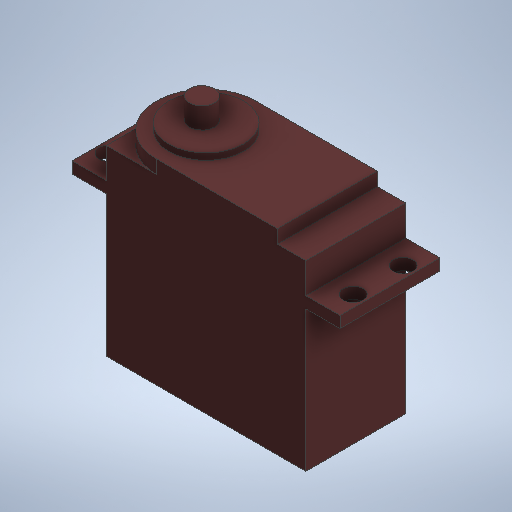
# Autodesk Inventor part: 996R모터
Saved by Autodesk Inventor 2025.2 (Build 292293000, 293)
## iProperties
Created: 2024-03-19
Part Number: 996R모터
Material: 일반
Document SubType Name: Modeling
Designer: USER
Density: 1 g/cm^3
Appearance: 기본값
Author: USER
## iProperties of the stored document 996R모터_3D 인쇄.ipt
Created: 2024-04-18
Part Number: 996R모터_3D 인쇄
Material: 일반
Document SubType Name: Modeling
Designer: USER
Density: 1 g/cm^3
Appearance: 기본값
Author: USER
Autodesk Inventor part; units mm, degrees
ref_plane "YZ Plane" through (0, 0, 0) normal (1, 0, 0) x (0, 1, 0)
ref_plane "XZ Plane" through (0, 0, 0) normal (0, 1, 0) x (-1, 0, 0)
ref_plane "XY Plane" through (0, 0, 0) normal (0, 0, 1) x (1, 0, 0)
sketch "스케치1" plane through (0, 0, 0) normal (0, 0, 1) x (1, 0, 0)
  line L0 (0, 0) -> (40, 0)
  line L1 (40, 0) -> (40, 36.6)
  line L2 (40, 36.6) -> (0, 36.6)
  line L3 (0, 36.6) -> (0, 0)
  dimension "d0" = 40
  dimension "d1" = 36.6
  constraints: 8 end point, 2 parallel, 1 horizontal, 1 perpendicular
  measures "d0" distance of L2.end L1.end
  measures "d1" distance of L0.end L1.end
extrude "돌출1" add sketch "스케치1" along normal blind 20
sketch "스케치2" plane through (0, 0, 20) normal (0, 0, 1) x (1, 0, 0)
  line L0 (40, 0) -> (40, 36.6) projected
  line L1 (40, 30.5) -> (46.85, 30.5)
  line L2 (46.85, 30.5) -> (46.85, 28.2)
  line L3 (46.85, 28.2) -> (40, 28.2)
  line L4 (40, 28.2) -> (40, 30.5)
  line L5 (0, 30.5) -> (-6.85, 30.5)
  line L6 (-6.85, 30.5) -> (-6.85, 28.2)
  line L7 (-6.85, 28.2) -> (0, 28.2)
  line L8 (0, 28.2) -> (0, 30.5)
  line L9 (0, 0) -> (40, 0) projected
  line L10 (0, 36.6) -> (0, 0) projected
  point P0 (40, 28.2)
  point P1 (0, 29.35)
  dimension "d4" = 6.85
  dimension "d5" = 6.85
  dimension "d6" = 2.3
  dimension "d7" = 2.3
  dimension "d8" = 30.5
  dimension "d9" = 30.5
  constraints: 16 end point, 4 parallel, 2 horizontal, 2 perpendicular, 2 point on line, 1 midpoint
  measures "d4" distance of L2.end L3.end
  measures "d5" distance of L7.end L6.end
  measures "d6" distance between parallel lines of L3 L1
  measures "d7" distance between parallel lines of L7 L5
  measures "d8" distance between parallel lines of L9 L1
  measures "d9" distance between parallel lines of L9 L5
extrude "돌출2" add sketch "스케치2" against normal blind 20
sketch "스케치3" plane through (0, 36.6, 0) normal (0, 1, 0) x (1, 0, 0)
  line L0 (40, 0) -> (0, 0) projected
  line L1 (0, 0) -> (0, -20) projected
  line L2 (40, -20) -> (0, -20) projected
  line L3 (40, 0) -> (40, -20) projected
  circle A0 centre (10, -10) radius 10
  line L4 (0, 0) -> (0, -20) projected
  line L5 (0, -20) -> (34.3, -20)
  line L6 (34.3, -20) -> (34.3, 0)
  line L7 (34.3, 0) -> (0, 0)
  line L8 (0, 0) -> (0, -20)
  line L9 (40, -20) -> (0, -20) projected
  point P0 (10, -20)
  point P1 (10, 0)
  dimension "d12" = 34.3
  constraints: 8 end point, 3 tangent, 2 parallel, 1 centre point, 1 horizontal, 1 perpendicular, 1 point on line
  measures "d12" distance of L7.end L6.end
extrude "돌출3" add sketch "스케치3" along normal blind 2.7 contours L6 L2 A0 L0 | A0
sketch "스케치4" plane through (0, 39.3, 0) normal (0, 1, 0) x (1, 0, 0)
  circle A0 centre (9.15, -10) radius 2.5
  arc A1 (10, 0) -> (10, -20) centre (10, -10) ccw projected
  line L0 (-6.85, -20) -> (-6.85, 0) projected
  point P0 (0, 0)
  point P1 (0, -10)
  point P2 (11.638, -9.755)
  point P3 (0, -10)
  point P4 (0, -10)
  dimension "d15" = 5
  dimension "d23" = 16
  constraints: 3 point on circle, 1 horizontal alignment, 3 other
  measures "d23" distance from line of L0 point (9.15, -10)
extrude "돌출4" add sketch "스케치4" along normal blind 5.5
sketch "스케치5" plane through (0, 39.3, 0) normal (0, 1, 0) x (1, 0, 0)
  circle A0 centre (9.15, -10) radius 2.5 projected
  line L0 (10, -20) -> (34.3, -20) projected
  line L1 (34.3, -20) -> (34.3, 0) projected
  line L2 (34.3, 0) -> (10, 0) projected
  arc A1 (10, 0) -> (10, -20) centre (10, -10) ccw projected
  circle A2 centre (10, -10) radius 7.5
  point P0 (0, 0)
  dimension "d20" = 15
  constraints: 1 centre point, 1 coincident
  measures "d20" diameter of A2
sketch "스케치6" plane through (0, 0, 20) normal (0, 0, 1) x (1, 0, 0)
  point P0 (0, 0)
extrude "돌출5" add sketch "스케치5" along normal blind 1.3 contours A2
sketch "스케치18" plane through (0, 39.3, 0) normal (0, 1, 0) x (1, 0, 0)
  point P0 (0, 0)
sketch "스케치19" plane through (40, 30.5, 20) normal (0, 1, 0) x (1, 0, 0)
  circle A0 centre (4.5, 15) radius 2
  circle A1 centre (4.5, 5) radius 2
  line L0 (6.85, 0) -> (0, 0) projected
  line L1 (6.85, 0) -> (6.85, 20) projected
  line L2 (0, 20) -> (6.85, 20) projected
  line L3 (0, 0) -> (0, 20) projected
  circle A2 centre (-30, 10) radius 7.5 projected
  line L4 (-30, 0) -> (-5.7, 0) projected
  line L5 (-5.7, 0) -> (-5.7, 20) projected
  line L6 (-5.7, 20) -> (-30, 20) projected
  arc A3 (-30, 20) -> (-30, 0) centre (-30, 10) ccw projected
  line L7 (-17.85, 0) -> (-17.85, 20)
  circle A4 centre (-44.5, 15) radius 2
  line L8 (-46.85, 0) -> (-46.85, 20) projected
  circle A5 centre (-44.5, 5) radius 2
  line L9 (-46.85, 20) -> (-40, 20) projected
  dimension "d24" = 4
  dimension "d25" = 4
  dimension "d26" = 10
  dimension "d27" = 5
  dimension "d29" = 2.35
  dimension "d30" = 4
  dimension "d31" = 2.35
  dimension "d32" = 2.35
  dimension "d33" = 4
  dimension "d34" = 2.35
  dimension "d35" = 10
  dimension "d36" = 5
  constraints: 4 centre point, 2 end point, 2 midpoint
  measures "d24" diameter of A0
  measures "d25" diameter of A1
  measures "d26" distance of A0.centre A1.centre
  measures "d27" distance from line of L2 A0.centre
  measures "d29" distance from line of L1 A0.centre
  measures "d30" diameter of A4
  measures "d31" distance from line of L8 A4.centre
  measures "d32" distance from line of L1 A1.centre
  measures "d33" diameter of A5
  measures "d34" distance from line of A5.centre L8
  measures "d35" distance of A4.centre A5.centre
  measures "d36" distance from line of L9 A4.centre
extrude "돌출6" cut sketch "스케치19" against normal through all contours A0 | A1 | A4 | A5
sketch "스케치35" plane through (0, 0, 0) normal (0, -1, 0) x (1, 0, 0)
  circle A0 centre (9.15, 10) radius 2.5 projected
  circle A1 centre (9.15, 10) radius 10.5
  point P0 (0, 0)
  dimension "d39" = 21
  constraints: 1 centre point, 1 coincident
  measures "d39" diameter of A1
sketch "스케치36" plane through (0, 0, 20) normal (0, 0, 1) x (1, 0, 0)
  line L0 (40, 0) -> (40, 28.2) projected
  line L1 (40, 28.2) -> (46.85, 28.2) projected
  line L2 (46.85, 28.2) -> (46.85, 30.5) projected
  line L3 (46.85, 30.5) -> (40, 30.5) projected
  line L4 (40, 30.5) -> (40, 36.6) projected
  line L5 (40, 36.6) -> (34.3, 36.6) projected
  line L6 (34.3, 36.6) -> (34.3, 39.3) projected
  line L7 (10, 39.3) -> (34.3, 39.3) projected
  line L8 (10, 36.6) -> (10, 39.3) projected
  line L9 (10, 36.6) -> (0, 36.6) projected
  line L10 (0, 36.6) -> (0, 30.5) projected
  line L11 (0, 30.5) -> (-6.85, 30.5) projected
  line L12 (-6.85, 30.5) -> (-6.85, 28.2) projected
  line L13 (-6.85, 28.2) -> (0, 28.2) projected
  line L14 (0, 28.2) -> (0, 0) projected
  line L15 (0, 0) -> (40, 0) projected
